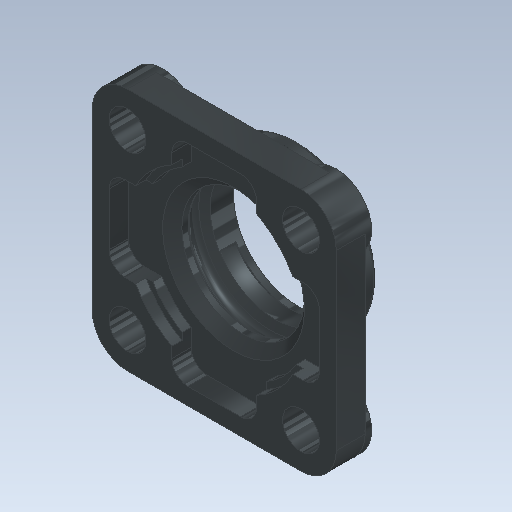
# Autodesk Inventor part: FY 503 M-housing
Saved by Autodesk Inventor 2020 (Build 240168000, 168)
## iProperties
Part Number: FY 503 M-housing
Material: Iron, Cast
Catalog Web Link: www.cadenas.de
Description: ayf_001hc_hh_hy-housing-Square flanged housings for Y-bearings
Vendor: SKF
Document SubType Name: Modeling
Designer: partserver
Manufacturer: SKF
Mass: 291.745 g
Surface Area: 192.771 cm^2
Volume: 40.8035 cm^3
Density: 7.15 g/cm^3
Appearance: Iron Gray
Category: PARTsolutions
Company: SKF
PSOL_IDENT_0: {$CADENAS_DATA\23d-libs\skf\bearings_units_and_housings\bearing_units\ball_bearing_units\y-units\y-b
PSOL_IDENT_1: earing_square_flanged_units_parts\ayf_001hc_hh_hy_housing.prj},196 {VTYP=3D},{NB=FY 503 M-housing},{
PSOL_IDENT_2: LINA=FY 503 M-housing},{NN=ayf_001hc_hh_hy-housing},{DATE=20.08.2020 13:45:19},{GEOMDATE=29.07.2020
PSOL_IDENT_3: 16:36:58},{VERSION=},{LINEID=8950},{WBVAR=COVER},{WBNUMERIC=}  {NB=FY 503 M-housing},{LINA=FY 503 M-
PSOL_IDENT_4: housing},{KT=DUMMY},{DESIGNATION=FY 503 M},{SS1=15.900},{T=32.900},{COVER=},{GN=1/4-28 SAE-LT},{D=40
PSOL_IDENT_5: .000},{DA=55.600},{DB1=50.000},{DB2=53.000},{DB=0.000},{A=26.000},{A1=11.000},{A2=17.000},{A3=3.200}
PSOL_IDENT_6: ,{A5=0.000},{J=54.000},{L=76.000},{N=11.500},{RG=1/4-28 UNF},{R1=19.000},{DN=6.500},{SWN=7.000},{J6=
PSOL_IDENT_7: 66.000},{J7=14.500},{N4=4.000},{EC=},{AEC=0.000},{DEC=0.000},{D1EC=0.000},{D2EC=0.000},{E=12},{DESIG
PSOL_IDENT_8: N=fy},{BRG=0.000},{ECPN=},{H4=MIN},{R2=MIN},{R3=MIN},{R4=MIN},{L1=MIN},{H5=MIN},{R5=MIN},{H6=MIN},{L
PSOL_IDENT_9: 2=MIN},{H7=MIN},{H8=MIN},{H9=MIN},{L3=MIN},{L4=MIN},{H10=MIN},{H11=MIN},{H12=MIN},{H13=MIN},{H14=MIN
PSOL_IDENT_10: },{R6=MIN},{L5=MIN},{H15=MIN},{H16=MIN},{SC=MIN}
NB: FY 503 M-housing
NN: ayf_001hc_hh_hy-housing
NT: Square flanged housings for Y-bearings
NBSYN: $DESIGNATION.$ECPN.-housing
LINA: FY 503 M-housing
CATALOG: SKF
DESIGNATION: FY 503 M
SS1: 15.9
T: 32.9
COVER: No End Cover
GN: 1/4-28 SAE-LT
D: 40
DA: 55.6
DB1: 50
DB2: 53
DB: 0
A: 26
A1: 11
A2: 17
A3: 3.2
A5: 0
J: 54
L: 76
N: 11.5
RG: 1/4-28 UNF
R1: 19
DN: 6.5
SWN: 7
J6: 66
J7: 14.5
N4: 4
AEC: 0
DEC: 0
D1EC: 0
D2EC: 0
DESIGN: fy
H4: 0
R2: 0
R3: 0
R4: 0
L1: 0
H5: 0
R5: 0
H6: 0
L2: 0
H7: 0
H8: 0
H9: 0
L3: 0
L4: 0
H10: 0
H11: 0
H12: 0
H13: 0
H14: 0
R6: 0
L5: 0
H15: 0
H16: 0
SC: 0
SUPPLIER: SKF
ARTICLENO: FY 503 M-housing
BOMINFO: FY 503 M-housing
CREATOR: CADENAS GmbH
Title: FY 503 M-housing
Author: Cadenas PARTsolutions
Comments: Square flanged housings for Y-bearings
Autodesk Inventor part; units mm, degrees
sketch "Sketch_1" plane through (0, 0, 0) normal (0, 0, 1) x (1, 0, 0)
  line L0 (0, 0) -> (0, 26)
  arc A0 (19.0788, 11) -> (19.0788, 23) centre (0, 17) ccw
  line L1 (19.0788, 11) -> (19.0788, 9)
  line L2 (19.0788, 9) -> (22.0788, 6)
  line L3 (22.0788, 6) -> (25.941, 6)
  line L4 (25.941, 6) -> (25.941, 3.2)
  line L5 (25.941, 3.2) -> (27.8, 3.2)
  line L6 (27.8, 3.2) -> (27.8, 0)
  line L7 (27.8, 0) -> (53.7401, 0)
  line L8 (53.7401, 0) -> (53.7401, 9)
  line L9 (53.7401, 9) -> (29.5, 9)
  arc A1 (26.5205, 11.6498) -> (29.5, 9) centre (29.5, 12) ccw
  line L10 (26.5205, 11.6498) -> (24.9897, 24.6751)
  arc A2 (24.9897, 24.6751) -> (23.5, 26) centre (23.5, 24.5) ccw
  line L11 (23.5, 26) -> (20, 26)
  line L12 (20, 26) -> (20, 23.9212)
  line L13 (20, 23.9212) -> (19.0788, 23)
  constraints: 28 end point, 6 point on circle, 3 centre point
revolve "Revolution1" add sketch "Sketch_1" angle 360 about axis through (0, 0, 0) along (0, -1, 0)
sketch "Sketch_2" plane through (0, 9, 0) normal (0, 1, 0) x (1, 0, 0)
  arc A0 (-34.7782, -19.2218) -> (-19.2218, -34.7782) centre (-27, -27) ccw
  line L0 (-19.2218, -34.7782) -> (-9.2696, -24.8259)
  arc A1 (-9.2696, -24.8259) -> (9.2696, -24.8259) centre (0, 0) ccw
  line L1 (9.2696, -24.8259) -> (19.2218, -34.7782)
  arc A2 (19.2218, -34.7782) -> (34.7782, -19.2218) centre (27, -27) ccw
  line L2 (34.7782, -19.2218) -> (24.8259, -9.2696)
  arc A3 (24.8259, -9.2696) -> (24.8259, 9.2696) centre (0, 0) ccw
  line L3 (24.8259, 9.2696) -> (34.7782, 19.2218)
  arc A4 (34.7782, 19.2218) -> (19.2218, 34.7782) centre (27, 27) ccw
  line L4 (19.2218, 34.7782) -> (9.2696, 24.8259)
  arc A5 (9.2696, 24.8259) -> (-9.2696, 24.8259) centre (0, 0) ccw
  line L5 (-9.2696, 24.8259) -> (-19.2218, 34.7782)
  arc A6 (-19.2218, 34.7782) -> (-34.7782, 19.2218) centre (-27, 27) ccw
  line L6 (-34.7782, 19.2218) -> (-24.8259, 9.2696)
  arc A7 (-24.8259, 9.2696) -> (-24.8259, -9.2696) centre (0, 0) ccw
  line L7 (-24.8259, -9.2696) -> (-34.7782, -19.2218)
  circle A8 centre (0, 0) radius 26
  constraints: 16 end point, 16 point on circle, 9 centre point
extrude "Extrusion1" add sketch "Sketch_2" along normal blind 2
sketch "Sketch_3" plane through (0, 0, 0) normal (0, 1, 0) x (-1, 0, 0)
  line L0 (76, -76) -> (76, 76)
  line L1 (76, 76) -> (-76, 76)
  line L2 (-76, 76) -> (-76, -76)
  line L3 (-76, -76) -> (76, -76)
  arc A0 (38, 27) -> (27, 38) centre (27, 27) ccw
  line L4 (27, 38) -> (-27, 38)
  arc A1 (-27, 38) -> (-38, 27) centre (-27, 27) ccw
  line L5 (-38, 27) -> (-38, -27)
  arc A2 (-38, -27) -> (-27, -38) centre (-27, -27) ccw
  line L6 (-27, -38) -> (27, -38)
  arc A3 (27, -38) -> (38, -27) centre (27, -27) ccw
  line L7 (38, -27) -> (38, 27)
  constraints: 16 end point, 8 point on circle, 4 centre point
extrude "Extrusion2" cut sketch "Sketch_3" along normal blind 26
sketch "Sketch4" plane through (-27, 0, -38) normal (0, -1, 0) x (1, 0, 0)
  point P0 (0, 65)
hole "Hole1" at (-27, 0, 27) direction (0, 1, 0) diameter 11.5 depth 11
pattern_linear "Rectangular Pattern1" count 2 spacing 54 along (1, 0, 0) count 2 spacing 54 along (0, 0, -1) of "Hole1"
sketch "Sketch_8" plane through (0, 0, 0) normal (1, 0, 0) x (0, 1, 0)
  line L0 (19, -25.6567) -> (16.6656, -5.7934)
  line L1 (16.6656, -5.7934) -> (19.8189, -5.4228)
  line L2 (19.8189, -5.4228) -> (22.1533, -25.2861)
  line L3 (22.1533, -25.2861) -> (19, -25.6567)
  line L4 (19, -25.6567) -> (16.6656, -5.7934)
  constraints: 10 end point
revolve "Revolution2" cut sketch "Sketch_8" angle 360 about axis through (0, 19, -25.6567) along (0, 0.1167192, -0.993165)
sketch "Sketch_6" plane through (0, 9, 0) normal (0, 1, 0) x (1, 0, 0)
  line L0 (-50, -14.5) -> (50, -14.5)
  arc A0 (-35, -14.5) -> (-31, -14.5) centre (-33, -14.5) ccw
  line L1 (-35, -14.5) -> (-31, -14.5)
  constraints: 4 end point, 2 point on circle, 1 centre point
revolve "Revolution3" cut sketch "Sketch_6" angle 360 about axis through (-50, 9, 14.5) along (-1, 0, 0)
sketch "Sketch_10" plane through (0, 0, 0) normal (0, 0, 1) x (1, 0, 0)
  line L0 (0, 3) -> (0, 29)
  line L1 (16, 21.0429) -> (16, 9.4959)
  line L2 (16, 9.4959) -> (22.25, 13.1043)
  arc A0 (22.25, 13.1043) -> (22.25, 17.4345) centre (21, 15.2694) ccw
  line L3 (22.25, 17.4345) -> (16, 21.0429)
  constraints: 8 end point, 2 point on circle, 1 centre point
revolve "Revolution4" cut sketch "Sketch_10" angle 360 about axis through (0, 3, 0) along (0, -1, 0)
sketch "Sketch_7" plane through (0, 17, 0) normal (0, 1, 0) x (1, 0, 0)
  arc A0 (-17.2017, 10.203) -> (-17.2017, -10.203) centre (0, 0) ccw
  line L0 (-17.2017, -10.203) -> (17.2017, -10.203)
  arc A1 (17.2017, -10.203) -> (17.2017, 10.203) centre (0, 0) ccw
  line L1 (17.2017, 10.203) -> (-17.2017, 10.203)
  constraints: 4 end point, 4 point on circle, 2 centre point
extrude "Extrusion3" cut sketch "Sketch_7" along normal blind 11.18
sketch "Sketch_11" plane through (0, 0, 0) normal (0, 1, 0) x (-1, 0, 0)
  arc A0 (32.75, 8.2) -> (27.75, 13.2) centre (27.75, 8.2) ccw
  line L0 (27.75, 13.2) -> (13.2, 13.2)
  line L1 (13.2, 13.2) -> (13.2, 27.75)
  arc A1 (13.2, 27.75) -> (8.2, 32.75) centre (8.2, 27.75) ccw
  line L2 (8.2, 32.75) -> (-8.2, 32.75)
  arc A2 (-8.2, 32.75) -> (-13.2, 27.75) centre (-8.2, 27.75) ccw
  line L3 (-13.2, 27.75) -> (-13.2, 13.2)
  line L4 (-13.2, 13.2) -> (-27.75, 13.2)
  arc A3 (-27.75, 13.2) -> (-32.75, 8.2) centre (-27.75, 8.2) ccw
  line L5 (-32.75, 8.2) -> (-32.75, -8.2)
  arc A4 (-32.75, -8.2) -> (-27.75, -13.2) centre (-27.75, -8.2) ccw
  line L6 (-27.75, -13.2) -> (-13.2, -13.2)
  line L7 (-13.2, -13.2) -> (-13.2, -27.75)
  arc A5 (-13.2, -27.75) -> (-8.2, -32.75) centre (-8.2, -27.75) ccw
  line L8 (-8.2, -32.75) -> (8.2, -32.75)
  arc A6 (8.2, -32.75) -> (13.2, -27.75) centre (8.2, -27.75) ccw
  line L9 (13.2, -27.75) -> (13.2, -13.2)
  line L10 (13.2, -13.2) -> (27.75, -13.2)
  arc A7 (27.75, -13.2) -> (32.75, -8.2) centre (27.75, -8.2) ccw
  line L11 (32.75, -8.2) -> (32.75, 8.2)
  constraints: 24 end point, 16 point on circle, 8 centre point
extrude "Extrusion4" cut sketch "Sketch_11" along normal blind 6
sketch "Sketch_12" plane through (0, 9, 0) normal (0, 1, 0) x (1, 0, 0)
  arc A0 (-36.5, 4.0095) -> (-36.2975, 3.807) centre (-36.2975, 4.0095) ccw
  line L0 (-36.2975, 3.807) -> (-34.9639, 3.807)
  arc A1 (-34.9639, 3.807) -> (-34.8207, 3.8663) centre (-34.9639, 4.0095) ccw
  line L1 (-34.8207, 3.8663) -> (-34.7661, 3.9209)
  arc A2 (-34.5522, 4.0095) -> (-34.7661, 3.9209) centre (-34.5522, 3.707) ccw
  line L2 (-34.5522, 4.0095) -> (-33.5464, 4.0095)
  arc A3 (-33.4032, 3.9502) -> (-33.5464, 4.0095) centre (-33.5464, 3.807) ccw
  line L3 (-33.4032, 3.9502) -> (-33.3193, 3.8663)
  arc A4 (-33.3193, 3.8663) -> (-33.1761, 3.807) centre (-33.1761, 4.0095) ccw
  line L4 (-33.1761, 3.807) -> (-32.045, 3.807)
  line L5 (-32.045, 3.807) -> (-32.045, 3.1793)
  line L6 (-32.045, 3.1793) -> (-33.26, 3.1793)
  arc A5 (-33.26, 3.1793) -> (-33.4625, 2.9768) centre (-33.26, 2.9767) ccw
  line L7 (-33.4625, 2.9768) -> (-33.4625, 1.6342)
  arc A6 (-33.5113, 1.5024) -> (-33.4625, 1.6342) centre (-33.665, 1.6342) ccw
  line L8 (-33.5113, 1.5024) -> (-34.6775, 0.1417)
  line L9 (-34.6775, 0.1417) -> (-35.2257, 0.6899)
  arc A7 (-35.285, 0.8331) -> (-35.2257, 0.6899) centre (-35.0825, 0.8331) ccw
  line L10 (-35.285, 0.8331) -> (-35.285, 2.3693)
  arc A8 (-35.285, 2.3693) -> (-35.4875, 2.5718) centre (-35.4875, 2.3692) ccw
  line L11 (-35.4875, 2.5718) -> (-36.2975, 2.5718)
  arc A9 (-36.2975, 2.5718) -> (-36.5, 2.3693) centre (-36.2975, 2.3692) ccw
  line L12 (-36.5, 2.3693) -> (-36.5, 0.6377)
  arc A10 (-36.5, 0.6377) -> (-36.432, 0.4863) centre (-36.2975, 0.6377) ccw
  line L13 (-36.432, 0.4863) -> (-34.6775, -1.0733)
  line L14 (-34.6775, -1.0733) -> (-36.2975, -1.0733)
  arc A11 (-36.2975, -1.0733) -> (-36.5, -1.2757) centre (-36.2975, -1.2758) ccw
  line L15 (-36.5, -1.2757) -> (-36.5, -2.8958)
  arc A12 (-36.5, -2.8958) -> (-36.2975, -3.0983) centre (-36.2975, -2.8957) ccw
  line L16 (-36.2975, -3.0983) -> (-34.9639, -3.0983)
  arc A13 (-34.9639, -3.0983) -> (-34.8207, -3.0389) centre (-34.9639, -2.8957) ccw
  line L17 (-34.8207, -3.0389) -> (-34.7368, -2.9551)
  arc A14 (-34.5936, -2.8958) -> (-34.7368, -2.9551) centre (-34.5936, -3.0983) ccw
  line L18 (-34.5936, -2.8958) -> (-33.7489, -2.8958)
  arc A15 (-33.6057, -2.9551) -> (-33.7489, -2.8958) centre (-33.7489, -3.0983) ccw
  line L19 (-33.6057, -2.9551) -> (-33.5218, -3.0389)
  arc A16 (-33.5218, -3.0389) -> (-33.3786, -3.0983) centre (-33.3786, -2.8957) ccw
  line L20 (-33.3786, -3.0983) -> (-32.045, -3.0983)
  line L21 (-32.045, -3.0983) -> (-32.045, -3.5032)
  line L22 (-32.045, -3.5032) -> (-34.475, -3.5032)
  arc A17 (-34.475, -3.5032) -> (-34.6775, -3.7058) centre (-34.475, -3.7058) ccw
  line L23 (-34.6775, -3.7058) -> (-34.6775, -6.9458)
  arc A18 (-34.88, -7.1483) -> (-34.6775, -6.9458) centre (-34.88, -6.9457) ccw
  line L24 (-34.88, -7.1483) -> (-35.69, -7.1483)
  arc A19 (-35.8925, -6.9458) -> (-35.69, -7.1483) centre (-35.69, -6.9457) ccw
  line L25 (-35.8925, -6.9458) -> (-35.8925, -6.1357)
  arc A20 (-35.69, -5.9333) -> (-35.8925, -6.1357) centre (-35.69, -6.1358) ccw
  line L26 (-35.69, -5.9333) -> (-35.4875, -5.9333)
  arc A21 (-35.4875, -5.9333) -> (-35.285, -5.7308) centre (-35.4875, -5.7307) ccw
  line L27 (-35.285, -5.7308) -> (-35.285, -4.3133)
  arc A22 (-35.285, -4.3133) -> (-35.4875, -4.1108) centre (-35.4875, -4.3133) ccw
  line L28 (-35.4875, -4.1108) -> (-36.2275, -4.1108)
  arc A23 (-36.2275, -4.1108) -> (-36.5, -4.3833) centre (-36.2275, -4.3833) ccw
  line L29 (-36.5, -4.3833) -> (-36.5, -8.7182)
  arc A24 (-36.5, -8.7182) -> (-36.2475, -8.9708) centre (-36.2475, -8.7183) ccw
  line L30 (-36.2475, -8.9708) -> (-34.2725, -8.9708)
  arc A25 (-34.2725, -8.9708) -> (-34.07, -8.7683) centre (-34.2725, -8.7682) ccw
  line L31 (-34.07, -8.7683) -> (-34.07, -5.5282)
  arc A26 (-33.8675, -5.3258) -> (-34.07, -5.5282) centre (-33.8675, -5.5283) ccw
  line L32 (-33.8675, -5.3258) -> (-32.45, -5.3258)
  arc A27 (-32.2475, -5.5282) -> (-32.45, -5.3258) centre (-32.45, -5.5283) ccw
  line L33 (-32.2475, -5.5282) -> (-32.2475, -7.5533)
  arc A28 (-32.45, -7.7557) -> (-32.2475, -7.5533) centre (-32.45, -7.5532) ccw
  line L34 (-32.45, -7.7557) -> (-33.26, -7.7557)
  arc A29 (-33.26, -7.7557) -> (-33.4625, -7.9582) centre (-33.26, -7.9583) ccw
  line L35 (-33.4625, -7.9582) -> (-33.4625, -9.3758)
  arc A30 (-33.4625, -9.3758) -> (-33.26, -9.5783) centre (-33.26, -9.3757) ccw
  line L36 (-33.26, -9.5783) -> (-31.8425, -9.5783)
  arc A31 (-31.8425, -9.5783) -> (-31.64, -9.3758) centre (-31.8425, -9.3757) ccw
  line L37 (-31.64, -9.3758) -> (-31.64, -3.7058)
  arc A32 (-31.64, -3.7058) -> (-31.8425, -3.5032) centre (-31.8425, -3.7058) ccw
  line L38 (-31.8425, -3.5032) -> (-31.8425, -3.0983)
  arc A33 (-31.8425, -3.0983) -> (-31.64, -2.8958) centre (-31.8425, -2.8957) ccw
  line L39 (-31.64, -2.8958) -> (-31.64, -1.2757)
  arc A34 (-31.64, -1.2757) -> (-31.8425, -1.0733) centre (-31.8425, -1.2758) ccw
  line L40 (-31.8425, -1.0733) -> (-33.4625, -1.0733)
  line L41 (-33.4625, -1.0733) -> (-31.6993, 0.6899)
  arc A35 (-31.6993, 0.6899) -> (-31.64, 0.8331) centre (-31.8425, 0.8331) ccw
  line L42 (-31.64, 0.8331) -> (-31.64, 2.9768)
  arc A36 (-31.64, 2.9768) -> (-31.8425, 3.1793) centre (-31.8425, 2.9767) ccw
  line L43 (-31.8425, 3.1793) -> (-31.8425, 3.807)
  arc A37 (-31.8425, 3.807) -> (-31.64, 4.0095) centre (-31.8425, 4.0095) ccw
  line L44 (-31.64, 4.0095) -> (-31.64, 5.6295)
  arc A38 (-31.64, 5.6295) -> (-31.8425, 5.832) centre (-31.8425, 5.6295) ccw
  line L45 (-31.8425, 5.832) -> (-33.26, 5.832)
  arc A39 (-33.26, 5.832) -> (-33.4625, 5.6295) centre (-33.26, 5.6295) ccw
  arc A40 (-33.665, 5.427) -> (-33.4625, 5.6295) centre (-33.665, 5.6295) ccw
  line L46 (-33.665, 5.427) -> (-33.8675, 5.427)
  arc A41 (-34.07, 5.6295) -> (-33.8675, 5.427) centre (-33.8675, 5.6295) ccw
  line L47 (-34.07, 5.6295) -> (-34.07, 6.3556)
  arc A42 (-34.0107, 6.4988) -> (-34.07, 6.3556) centre (-33.8675, 6.3556) ccw
  line L48 (-34.0107, 6.4988) -> (-33.9268, 6.5827)
  arc A43 (-33.9268, 6.5827) -> (-33.8675, 6.7259) centre (-34.07, 6.7259) ccw
  line L49 (-33.8675, 6.7259) -> (-33.8675, 8.0595)
  arc A44 (-33.8675, 8.0595) -> (-34.07, 8.262) centre (-34.07, 8.0595) ccw
  line L50 (-34.07, 8.262) -> (-34.6775, 8.262)
  arc A45 (-34.6775, 8.262) -> (-34.88, 8.0595) centre (-34.6775, 8.0595) ccw
  line L51 (-34.88, 8.0595) -> (-34.88, 6.7259)
  arc A46 (-34.88, 6.7259) -> (-34.8207, 6.5827) centre (-34.6775, 6.7259) ccw
  line L52 (-34.8207, 6.5827) -> (-34.7368, 6.4988)
  arc A47 (-34.6775, 6.3556) -> (-34.7368, 6.4988) centre (-34.88, 6.3556) ccw
  line L53 (-34.6775, 6.3556) -> (-34.6775, 5.6295)
  arc A48 (-34.88, 5.427) -> (-34.6775, 5.6295) centre (-34.88, 5.6295) ccw
  line L54 (-34.88, 5.427) -> (-35.59, 5.427)
  arc A49 (-35.8925, 5.7295) -> (-35.59, 5.427) centre (-35.59, 5.7295) ccw
  line L55 (-35.8925, 5.7295) -> (-35.8925, 7.452)
  arc A50 (-35.69, 7.6545) -> (-35.8925, 7.452) centre (-35.69, 7.452) ccw
  line L56 (-35.69, 7.6545) -> (-35.4875, 7.6545)
  arc A51 (-35.4875, 7.6545) -> (-35.285, 7.857) centre (-35.4875, 7.857) ccw
  line L57 (-35.285, 7.857) -> (-35.285, 9.882)
  arc A52 (-35.285, 9.882) -> (-35.4875, 10.0845) centre (-35.4875, 9.882) ccw
  line L58 (-35.4875, 10.0845) -> (-36.2975, 10.0845)
  arc A53 (-36.2975, 10.0845) -> (-36.5, 9.882) centre (-36.2975, 9.882) ccw
  line L59 (-36.5, 9.882) -> (-36.5, 4.0095)
  constraints: 120 end point, 108 point on circle, 54 centre point
extrude "Extrusion5" add sketch "Sketch_12" along normal blind 0.7
ref_plane "brg_XY" through (0, 17, 0) normal (0, 1, 0) x (1, 0, 0)
ref_plane "brg_YZ" through (0, 17, 0) normal (1, 0, 0) x (0, 0, -1)
ref_plane "brg_ZX" through (0, 17, 0) normal (0, 0, -1) x (0, 1, 0)
ref_plane "gn_XY" through (0, 19, -25.6567) normal (1, 0, 0) x (0, 0.9848078, 0.1736482)
ref_plane "gn_YZ" through (0, 19, -25.6567) normal (0, 0.9848078, 0.1736482) x (0, -0.1736482, 0.9848078)
ref_plane "gn_ZX" through (0, 19, -25.6567) normal (0, -0.1736482, 0.9848078) x (1, 0, 0)
ref_plane "housing_XY" through (0, 0, 0) normal (0, 1, 0) x (1, 0, 0)
ref_plane "housing_YZ" through (0, 0, 0) normal (1, 0, 0) x (0, 0, -1)
ref_plane "housing_ZX" through (0, 0, 0) normal (0, 0, -1) x (0, 1, 0)
body "Solid1"
